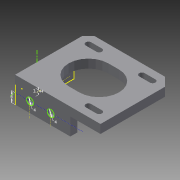
# Autodesk Inventor part: bart Y motor mount v2
Saved by Autodesk Inventor 2014 SP1 (Build 180222100, 222)
## iProperties
Created: 2015-07-22
Part Number: bart Y motor mount v2
Material: Generic
Document SubType Name: Modeling
Designer: Mon
Density: 1 g/cm^3
Appearance: Default
Author: Mon
Autodesk Inventor part; units mm, degrees
ref_plane "YZ Plane" through (0, 0, 0) normal (1, 0, 0) x (0, 1, 0)
ref_plane "XZ Plane" through (0, 0, 0) normal (0, 1, 0) x (-1, 0, 0)
ref_plane "XY Plane" through (0, 0, 0) normal (0, 0, 1) x (1, 0, 0)
sketch "Sketch2" plane through (0, 0, 0) normal (0, 0, 1) x (1, 0, 0)
  line L0 (49.4803, 37.44) -> (44.4803, 42.44)
  line L1 (5.7803, 38.32) -> (5.3662, 38.2655)
  line L2 (4.9803, 38.1056) -> (4.6489, 37.8514)
  line L3 (3.4803, 42.44) -> (44.4803, 42.44)
  line L4 (-0.0197, 38.94) -> (3.4803, 42.44)
  line L5 (-0.0197, 0) -> (49.4803, 0)
  line L6 (49.4803, 37.44) -> (49.4803, 0)
  line L7 (4.2348, 36.3059) -> (4.3946, 35.92)
  line L8 (10.1721, 18.2436) -> (11.321, 15.47)
  line L9 (35.2348, 6.1341) -> (35.1803, 5.72)
  line L10 (4.6489, 35.5886) -> (4.9803, 35.3344)
  line L11 (36.7803, 38.32) -> (36.3662, 38.2655)
  line L12 (36.3662, 35.1745) -> (36.7803, 35.12)
  line L13 (35.3946, 35.92) -> (35.6489, 35.5886)
  line L14 (35.1803, 36.72) -> (35.2348, 36.3059)
  line L15 (35.2348, 5.3059) -> (35.3946, 4.92)
  line L16 (21.2803, 32.72) -> (18.3039, 32.3281)
  line L17 (35.2348, 37.1341) -> (35.1803, 36.72)
  line L18 (35.3946, 6.52) -> (35.2348, 6.1341)
  line L19 (35.9803, 7.1056) -> (35.6489, 6.8514)
  line L20 (36.7803, 7.32) -> (36.3662, 7.2655)
  line L21 (35.6489, 6.8514) -> (35.3946, 6.52)
  line L22 (35.9803, 35.3344) -> (36.3662, 35.1745)
  line L23 (4.6489, 37.8514) -> (4.3946, 37.52)
  line L24 (5.3662, 38.2655) -> (4.9803, 38.1056)
  line L25 (4.3946, 35.92) -> (4.6489, 35.5886)
  line L26 (35.6489, 35.5886) -> (35.9803, 35.3344)
  line L27 (36.3662, 38.2655) -> (35.9803, 38.1056)
  line L28 (5.3662, 35.1745) -> (5.7803, 35.12)
  line L29 (4.9803, 35.3344) -> (5.3662, 35.1745)
  line L30 (4.1803, 36.72) -> (4.2348, 36.3059)
  line L31 (4.2348, 37.1341) -> (4.1803, 36.72)
  line L32 (4.3946, 37.52) -> (4.2348, 37.1341)
  line L33 (18.3039, 10.1119) -> (21.2803, 9.72)
  line L34 (15.5303, 11.2607) -> (18.3039, 10.1119)
  line L35 (13.1485, 13.0883) -> (15.5303, 11.2607)
  line L36 (11.321, 15.47) -> (13.1485, 13.0883)
  line L37 (9.7803, 21.22) -> (10.1721, 18.2436)
  line L38 (10.1721, 24.1964) -> (9.7803, 21.22)
  line L39 (11.321, 26.97) -> (10.1721, 24.1964)
  line L40 (13.1485, 29.3517) -> (11.321, 26.97)
  line L41 (15.5303, 31.1793) -> (13.1485, 29.3517)
  line L42 (18.3039, 32.3281) -> (15.5303, 31.1793)
  line L43 (36.3662, 7.2655) -> (35.9803, 7.1056)
  line L44 (36.3662, 4.1745) -> (36.7803, 4.12)
  line L45 (35.9803, 4.3344) -> (36.3662, 4.1745)
  line L46 (35.6489, 4.5886) -> (35.9803, 4.3344)
  line L47 (35.3946, 4.92) -> (35.6489, 4.5886)
  line L48 (35.1803, 5.72) -> (35.2348, 5.3059)
  line L49 (35.2348, 36.3059) -> (35.3946, 35.92)
  line L50 (35.3946, 37.52) -> (35.2348, 37.1341)
  line L51 (35.6489, 37.8514) -> (35.3946, 37.52)
  line L52 (35.9803, 38.1056) -> (35.6489, 37.8514)
  line L53 (27.4803, 9.72) -> (30.4567, 10.1119)
  line L54 (35.612, 29.3517) -> (33.2303, 31.1793)
  line L55 (38.5884, 24.1964) -> (37.4396, 26.97)
  line L56 (12.7803, 35.3344) -> (13.1116, 35.5886)
  line L57 (30.4567, 10.1119) -> (33.2303, 11.2607)
  line L58 (38.9803, 21.22) -> (38.5884, 24.1964)
  line L59 (43.7803, 35.3344) -> (44.1116, 35.5886)
  line L60 (44.5257, 6.1341) -> (44.3659, 6.52)
  line L61 (38.5884, 18.2436) -> (38.9803, 21.22)
  line L62 (44.3659, 37.52) -> (44.1116, 37.8514)
  line L63 (44.1116, 37.8514) -> (43.7803, 38.1056)
  line L64 (13.3659, 35.92) -> (13.5258, 36.3059)
  line L65 (44.1116, 4.5886) -> (44.3659, 4.92)
  line L66 (43.3944, 38.2655) -> (42.9803, 38.32)
  line L67 (30.4567, 32.3281) -> (27.4803, 32.72)
  line L68 (44.1116, 35.5886) -> (44.3659, 35.92)
  line L69 (35.612, 13.0883) -> (37.4396, 15.47)
  line L70 (37.4396, 26.97) -> (35.612, 29.3517)
  line L71 (37.4396, 15.47) -> (38.5884, 18.2436)
  line L72 (43.7803, 4.3344) -> (44.1116, 4.5886)
  line L73 (13.1116, 37.8514) -> (12.7803, 38.1056)
  line L74 (33.2303, 31.1793) -> (30.4567, 32.3281)
  line L75 (12.7803, 38.1056) -> (12.3944, 38.2655)
  line L76 (44.3659, 6.52) -> (44.1116, 6.8514)
  line L77 (33.2303, 11.2607) -> (35.612, 13.0883)
  line L78 (42.9803, 4.12) -> (43.3944, 4.1745)
  line L79 (44.5257, 37.1341) -> (44.3659, 37.52)
  line L80 (43.7803, 7.1056) -> (43.3944, 7.2655)
  line L81 (44.5257, 5.3059) -> (44.5803, 5.72)
  line L82 (43.7803, 38.1056) -> (43.3944, 38.2655)
  line L83 (12.3944, 38.2655) -> (11.9803, 38.32)
  line L84 (44.3659, 35.92) -> (44.5257, 36.3059)
  line L85 (43.3944, 35.1745) -> (43.7803, 35.3344)
  line L86 (43.3944, 4.1745) -> (43.7803, 4.3344)
  line L87 (13.1116, 35.5886) -> (13.3659, 35.92)
  line L88 (11.9803, 35.12) -> (12.3944, 35.1745)
  line L89 (42.9803, 35.12) -> (43.3944, 35.1745)
  line L90 (44.5803, 5.72) -> (44.5257, 6.1341)
  line L91 (43.3944, 7.2655) -> (42.9803, 7.32)
  line L92 (13.5258, 36.3059) -> (13.5803, 36.72)
  line L93 (44.3659, 4.92) -> (44.5257, 5.3059)
  line L94 (13.5258, 37.1341) -> (13.3659, 37.52)
  line L95 (44.5803, 36.72) -> (44.5257, 37.1341)
  line L96 (44.5257, 36.3059) -> (44.5803, 36.72)
  line L97 (13.3659, 37.52) -> (13.1116, 37.8514)
  line L98 (44.1116, 6.8514) -> (43.7803, 7.1056)
  line L99 (12.3944, 35.1745) -> (12.7803, 35.3344)
  line L100 (13.5803, 36.72) -> (13.5258, 37.1341)
  line L101 (5.7803, 38.32) -> (11.9803, 38.32)
  line L102 (5.7803, 35.12) -> (11.9803, 35.12)
  line L103 (36.7803, 35.12) -> (42.9803, 35.12)
  line L104 (36.7803, 7.32) -> (42.9803, 7.32)
  line L105 (36.7803, 4.12) -> (42.9803, 4.12)
  line L106 (21.2803, 32.72) -> (27.4803, 32.72)
  line L107 (21.2803, 9.72) -> (27.4803, 9.72)
  line L108 (36.7803, 38.32) -> (42.9803, 38.32)
  line L109 (-0.0197, 0) -> (-0.0197, 38.94)
  point P0 (0, 0)
  constraints: 220 end point
extrude "Extrusion1" add sketch "Sketch2" along normal blind 5
sketch "Sketch3" plane through (0, 0, 0) normal (0, 0, -1) x (-1, 0, 0)
  line L0 (0, 0) -> (-4, 0)
  line L1 (-4, 0) -> (-4, 30)
  line L2 (-4, 30) -> (0, 30)
  line L3 (0, 30) -> (0, 0)
  dimension "d2" = 4
  dimension "d3" = 30
  constraints: 8 end point, 2 parallel, 1 horizontal, 1 perpendicular
  measures "d2" distance of L1.end L2.end
  measures "d3" distance of L0.end L1.end
extrude "Extrusion2" add sketch "Sketch3" along normal blind 10
sketch "Sketch4" plane through (0, 0, 0) normal (0, 0, -1) x (-1, 0, 0)
  line L0 (-4, 0) -> (-32, 0)
  line L1 (-32, 0) -> (-32, 4)
  line L2 (-32, 4) -> (-4, 4)
  line L3 (-4, 4) -> (-4, 0)
  dimension "d6" = 28
  dimension "d7" = 4
  constraints: 8 end point, 2 parallel, 1 horizontal, 1 perpendicular
  measures "d6" distance of L1.end L2.end
  measures "d7" distance of L0.end L1.end
extrude "Extrusion3" add sketch "Sketch4" along normal blind 10
sketch "Sketch5" plane through (0, 0, 0) normal (-1, 0, 0) x (0, 0, 1)
  line L0 (0, 30) -> (0, 0) projected
  line L1 (0, 30) -> (-10, 30) projected
  line L2 (-10, 0) -> (-10, 30) projected
  line L3 (0, 0) -> (-10, 0) projected
  line L4 (-12.7767, 12.5) -> (11.2598, 12.5)
  line L5 (-4, 28.2185) -> (-4, -2.7903)
  constraints: 4 end point, 1 parallel, 1 perpendicular
hole "Hole1" at (0, 7.828, -4) direction (1, 0, 0) diameter 4 end through all
hole "Hole2" at (0, 18.6411, -4.0242) direction (1, 0, 0) diameter 4 end through all
sketch "Sketch14" plane through (0, 0, -10) normal (0, -1, 0) x (1, 0, 0)
  line L0 (0, 10) -> (0, 0) projected
  line L1 (0, 0) -> (0, 6) construction
  line L2 (0, 6) -> (39.6978, 6) construction
  line L3 (8.5455, 8.0526) -> (8.5455, -2.848) construction
  line L4 (20.5377, 7.5413) -> (20.5377, -0.9308) construction
  circle A0 centre (8.5455, 6) radius 2
  circle A1 centre (20.5377, 6) radius 2
  dimension "d70" = 6
  dimension "d71" = 4
  dimension "d74" = 4
  constraints: 8 end point, 5 point on line, 2 centre point, 2 perpendicular, 1 parallel
  measures "d70" distance of L0.end L1.end
  measures "d71" diameter of A0
  measures "d74" diameter of A1
hole "Hole5" at (8.5455, 0, -4) direction (0, 1, 0) diameter 4 end through all
extrude "Extrusion11" cut sketch "Sketch14" against normal through all contours A1
sketch "Sketch15" plane through (4, 30, 0) normal (1, 0, 0) x (0, 0, -1)
  circle A0 centre (4.0242, -11.3589) radius 2 projected
  line L0 (3.9946, -14.2505) -> (1.5052, -12.7791)
  line L1 (1.5052, -12.7791) -> (1.5348, -9.8875)
  line L2 (1.5348, -9.8875) -> (4.0538, -8.4673)
  line L3 (4.0538, -8.4673) -> (6.5431, -9.9388)
  line L4 (6.5431, -9.9388) -> (6.5135, -12.8304)
  line L5 (6.5135, -12.8304) -> (3.9946, -14.2505)
  point P0 (0, -30)
  constraints: 12 end point, 1 coincident, 13 other
extrude "Extrusion12" cut sketch "Sketch15" against normal blind 2
sketch "Sketch16" plane through (4, 30, 0) normal (1, 0, 0) x (0, 0, -1)
  circle A0 centre (4, -22.172) radius 2 projected
  line L0 (0, -26) -> (0, 0) projected
  line L1 (6.5135, -12.8304) -> (6.5135, -28.1931) construction
  line L2 (6.5135, -23.6354) -> (3.9894, -25.0805)
  line L3 (3.9894, -25.0805) -> (1.4759, -23.6171)
  line L4 (1.4759, -23.6171) -> (1.4865, -20.7086)
  line L5 (1.4865, -20.7086) -> (4.0106, -19.2635)
  line L6 (4.0106, -19.2635) -> (6.5241, -20.7269)
  line L7 (6.5241, -20.7269) -> (6.5135, -23.6354)
  point P0 (0, -30)
  constraints: 14 end point, 1 coincident, 1 parallel, 1 point on line, 13 other
extrude "Extrusion13" cut sketch "Sketch16" against normal blind 2
sketch "Sketch17" plane through (4, 4, 0) normal (0, 1, 0) x (1, 0, 0)
  circle A0 centre (4.5455, 4) radius 2 projected
  line L0 (8.217, 4) -> (6.3812, 0.8204)
  line L1 (6.3812, 0.8204) -> (2.7097, 0.8204)
  line L2 (2.7097, 0.8204) -> (0.8739, 4)
  line L3 (0.8739, 4) -> (2.7097, 7.1796)
  line L4 (2.7097, 7.1796) -> (6.3812, 7.1796)
  line L5 (6.3812, 7.1796) -> (8.217, 4)
  point P0 (-4, 0)
  constraints: 12 end point, 1 coincident, 13 other
extrude "Extrusion14" cut sketch "Sketch17" against normal blind 2
sketch "Sketch18" plane through (4, 4, 0) normal (0, 1, 0) x (1, 0, 0)
  circle A0 centre (16.5377, 4) radius 2 projected
  line L0 (20.1924, 4) -> (18.365, 0.8349)
  line L1 (18.365, 0.8349) -> (14.7103, 0.8349)
  line L2 (14.7103, 0.8349) -> (12.8829, 4)
  line L3 (12.8829, 4) -> (14.7103, 7.1651)
  line L4 (14.7103, 7.1651) -> (18.365, 7.1651)
  line L5 (18.365, 7.1651) -> (20.1924, 4)
  point P0 (-4, 0)
  constraints: 12 end point, 1 coincident, 13 other
extrude "Extrusion15" cut sketch "Sketch18" against normal blind 2
sketch "Sketch19" plane through (4, 30, 0) normal (1, 0, 0) x (0, 0, -1)
  line L0 (6.5241, -20.7269) -> (6.5135, -23.6354) projected
  line L1 (6.5135, -23.6354) -> (3.9894, -25.0805) projected
  line L2 (3.9894, -25.0805) -> (1.4759, -23.6171) projected
  line L3 (1.4759, -23.6171) -> (1.4865, -20.7086) projected
  line L4 (1.4865, -20.7086) -> (4.0106, -19.2635) projected
  line L5 (4.0106, -19.2635) -> (6.5241, -20.7269) projected
  line L6 (6.5135, -12.8304) -> (3.9946, -14.2505) projected
  line L7 (3.9946, -14.2505) -> (1.5052, -12.7791) projected
  line L8 (1.5052, -12.7791) -> (1.5348, -9.8875) projected
  line L9 (1.5348, -9.8875) -> (4.0538, -8.4673) projected
  line L10 (4.0538, -8.4673) -> (6.5431, -9.9388) projected
  line L11 (6.5431, -9.9388) -> (6.5135, -12.8304) projected
  line L12 (0, -26) -> (10, -26) projected
  line L13 (10, 0) -> (10, -26) projected
  line L14 (0, 0) -> (10, 0) projected
  line L15 (0, -26) -> (0, 0) projected
  line L16 (4.0538, -22.1628) -> (7.7978, -22.1628) construction
  line L17 (7.7978, -22.1628) -> (7.7978, -2.0426) construction
  point P0 (0, -30)
  dimension "d92" = 3.744
  constraints: 4 end point, 2 perpendicular
  measures "d92" distance of L16.start L16.end
body "Solid1"
